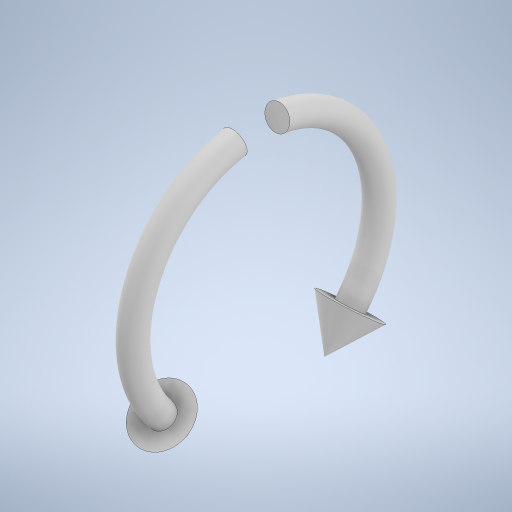
# Autodesk Inventor part: Turns
Saved by Autodesk Inventor 2023 (Build 270158000, 158)
## iProperties
Created: 2022-10-18
Part Number: Turns
Material: Generic
Document SubType Name: Modeling
Designer: benni
Density: 1 g/cm^3
Appearance: Default
Author: benni
Autodesk Inventor part; units mm, degrees
ref_plane "YZ Plane" through (0, 0, 0) normal (1, 0, 0) x (0, 1, 0)
ref_plane "XZ Plane" through (0, 0, 0) normal (0, 1, 0) x (-1, 0, 0)
ref_plane "XY Plane" through (0, 0, 0) normal (0, 0, 1) x (1, 0, 0)
sketch "Sketch1" plane through (0, 0, 0) normal (0, 0, 1) x (1, 0, 0)
  line L0 (0, 0) -> (7, 0)
  circle A0 centre (0, 10) radius 1
  dimension "d0" = 7
  dimension "d2" = 2
  dimension "d3" = 10
  constraints: 2 end point, 1 centre point, 1 horizontal
  measures "d0" distance of L0.start L0.end
  measures "d2" diameter of A0
  measures "d3" distance of L0.start A0.centre
revolve "Revolution1" add sketch "Sketch1" angle 260 mid plane about axis through (0, 0, 0) along (1, 0, 0)
revolve "Revolution2" cut sketch "Sketch1" angle 20 mid plane about axis through (0, 0, 0) along (1, 0, 0)
sketch "Sketch2" plane through (0, 0, 0) normal (1, 0, 0) x (0, 1, 0)
  line L0 (-7.0707, 8.4265) -> (-5.7851, 6.8944) projected
  line L1 (-6.4279, 7.6604) -> (-11.6539, 3.2753)
  line L2 (-6.4279, 7.6604) -> (-7.9026, 9.418)
  line L3 (-7.9026, 9.418) -> (-8.9379, 5.5543)
  point P0 (0, 0)
  dimension "d6" = 35
  dimension "d8" = 4
  constraints: 6 end point, 1 midpoint, 1 perpendicular, 1 point on line
  measures "d6" angle of L1 L3
  measures "d8" distance of L2.end L3.end
revolve "Revolution3" add sketch "Sketch2" angle 360 about axis through (0, -6.4279, 7.6604) along (0, 0.7660444, 0.6427876)
sketch "Sketch3" plane through (0, 0, 0) normal (1, 0, 0) x (0, 1, 0)
  line L0 (-7.0707, -8.4265) -> (-5.7851, -6.8944) projected
  line L1 (-6.4279, -7.6604) -> (-9.9209, -4.7295)
  line L2 (-6.4279, -7.6604) -> (-7.9026, -9.418)
  line L3 (-7.9026, -9.418) -> (-8.9379, -5.5543)
  point P0 (0, 0)
  dimension "d10" = 35
  dimension "d11" = 0
  dimension "d12" = 4
  constraints: 6 end point, 1 midpoint, 1 point on line
  measures "d10" angle of L3 L1
  measures "d11" distance between parallel lines of L0 L2
  measures "d12" distance of L2.end L3.end
revolve "Revolution4" add sketch "Sketch3" angle 360 about axis through (0, -6.4279, -7.6604) along (0, 0.7660444, -0.6427876)
body "Solid1"
